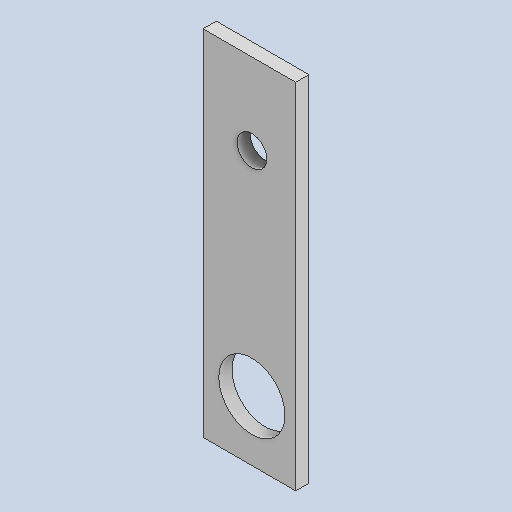
# Autodesk Inventor part: backWheelNoMotor brake mount
Saved by Autodesk Inventor 2022.2 (Build 262287000, 287)
## iProperties
Created: 2022-04-04
Part Number: backWheelNoMotor brake mount
Material: Generic
Document SubType Name: Sheet Metal
Designer: foriw
Density: 1 g/cm^3
Sheet Metal Rule: Default_mm
Appearance: Default
Author: foriw
Autodesk Inventor part; units mm, degrees
ref_plane "YZ Plane" through (0, 0, 0) normal (1, 0, 0) x (0, 1, 0)
ref_plane "XZ Plane" through (0, 0, 0) normal (0, 1, 0) x (-1, 0, 0)
ref_plane "XY Plane" through (0, 0, 0) normal (0, 0, 1) x (1, 0, 0)
sketch "Sketch1" plane through (0, 0, 0) normal (0, 0, 1) x (1, 0, 0)
  line L0 (0, 33.4599) -> (-14, 33.4599) projected
  line L1 (0, 0) -> (-14, 0) projected
  line L2 (0, 0) -> (-14, 0)
  line L3 (-14, 0) -> (-14, 33.4599)
  line L4 (-14, 33.4599) -> (0, 33.4599)
  line L5 (0, 33.4599) -> (0, 0)
  line L6 (-14, 33.4599) -> (0, 33.4599)
  line L7 (0, 33.4599) -> (0, 53.4599)
  line L8 (0, 53.4599) -> (-14, 53.4599)
  line L9 (-14, 53.4599) -> (-14, 33.4599)
  dimension "d0" = 20
  constraints: 16 end point, 4 parallel, 2 horizontal, 2 perpendicular, 1 point on line
  measures "d0" distance of L7.end L6.end
extrude "Extrusion1" add sketch "Sketch1" along normal blind 2
sketch "Sketch2" plane through (0, 0, 2) normal (0, 0, 1) x (1, 0, 0)
  circle A0 centre (-7.2474, 41.2065) radius 6.15 projected
  circle A1 centre (-7.2474, 41.2065) radius 2.15 projected
  circle A2 centre (-6.6223, 9.0626) radius 17.5 projected
  circle A3 centre (-6.6223, 9.0626) radius 5 projected
  circle A4 centre (-6.6223, 9.0626) radius 32.15
  circle A5 centre (-6.6223, 41.2126) radius 2.25
  line L0 (-6.6223, 9.0626) -> (-6.6223, 22.3742) construction
  line L1 (-6.6223, 41.2126) -> (-6.6223, 9.0626) construction
  circle A6 centre (-6.6223, 9.0626) radius 5 projected
  circle A7 centre (-6.6223, 9.0626) radius 5 projected
  point P0 (0, 0)
  dimension "d3" = 4.5
  dimension "d4" = 0
  constraints: 4 end point, 2 centre point, 2 point on circle, 1 coincident, 1 vertical
  measures "d3" diameter of A5
  measures "d4" distance between parallel lines of L1 L0
extrude "Extrusion2" cut sketch "Sketch2" against normal through all contours A5 A1 A4 | A4 A1 A5 | A1 A4 A5 | A5 A4 A1 | A3 picked at (-4.7487, 40.4928) picked at (-4.8145, 41.5313) picked at (-6.9297, 41.9074) picked at (-6.9194, 40.5049)
equation "\"BendRadius\" = Thickness"
equation "\"BendReliefWidth\" = Thickness"
equation "\"BendReliefDepth\" = 0.5 * Thickness"
equation "\"CornerReliefSize\" = 4 * Thickness"
equation "\"MinimumRemnant\" = 2 * Thickness"
equation "\"TransitionRadius\" = BendRadius"
equation "\"JacobiRadiusSize\" = BendRadius"
equation "\"GapSize\" = Thickness"
equation "\"Thickness\" = 2"
body "Solid1"
